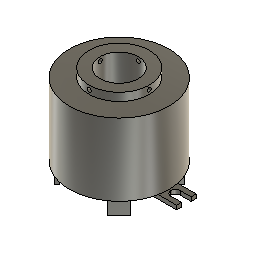
static base (Autodesk Fusion 360 archive; units mm, degrees)
design "slipring model"
Autodesk Fusion 360 part; units mm, degrees
sketch "Sketch1" plane through (0, 0, 0) normal (0, 0, 1) x (1, 0, 0)
  line L0 (36.0002, -9.75) -> (67.0101, -9.75)
  line L1 (67.0002, 9.75) -> (36.0002, 9.75)
  line L2 (67.0101, -4.75) -> (56.25, -4.75)
  arc A0 (56.25, 4.75) -> (51.5, 0) centre (56.25, 0) ccw
  line L3 (67.0101, -4.75) -> (67.0101, -9.75)
  line L4 (36.0002, 9.75) -> (36.0002, -9.75)
  arc A1 (51.5, 0) -> (56.25, -4.75) centre (56.25, 0) ccw
  line L5 (56.25, 4.75) -> (67.0002, 4.75)
  line L6 (67.0002, 4.75) -> (67.0002, 9.75)
  line L7 (0, 0) -> (36.0002, 0)
  point P0 (51.5001, 4.75)
  dimension "d7" = 4.75
  dimension "d8" = 4.75
  dimension "d9" = 4.75
  dimension "d10" = 31
  dimension "d11" = 19.5
  constraint perpendicular L5 L6
  constraint perpendicular L2 L3
  constraint tangent L2 A1
  constraint coincident P0 L5
  constraint tangent A0 L5
  constraint perpendicular L1 L6
  constraint perpendicular L1 L4
  constraint perpendicular L0 L3
  constraint coincident L7.start origin
  constraint midpoint L4 L7.end
  measures "d7" distance of A0.end P0
  measures "d8" radius of A1
  measures "d9" radius of A0
  measures "d10" distance of L1.start L1.end
  measures "d11" distance of L1.end L0.start
extrude "Extrude1" add sketch "Sketch1" along normal blind 4
sketch "Sketch2" plane through (0, 0, 4) normal (0, 0, 1) x (-1, 0, 0)
  line L0 (-56.25, -4.75) -> (-67.0002, -4.75)
  line L1 (-67.0002, -4.75) -> (-67.0002, -9.75)
  line L2 (-67.0101, 9.75) -> (-67.0101, 4.75)
  line L3 (-67.0101, 4.75) -> (-56.25, 4.75)
  arc A0 (-51.5, 0) -> (-56.25, 4.75) centre (-56.25, 0) ccw
  arc A1 (-56.25, -4.75) -> (-51.5, 0) centre (-56.25, 0) ccw
  circle A2 centre (0, 0) radius 49.5
  circle A3 centre (0, 0) radius 19.05
  dimension "d14" = 99
  dimension "d15" = 38.1
  constraint coincident A2.centre A3.centre
  measures "d14" diameter of A2
  measures "d15" diameter of A3
extrude "Extrude2" add sketch "Sketch2" along normal blind 72
sketch "Sketch3" plane through (0, 0, 76) normal (0, 0, 1) x (-1, 0, 0)
  circle A0 centre (0, 0) radius 19.05
  circle A1 centre (0, 0) radius 49.5
  circle A2 centre (0, 0) radius 19.05
  circle A3 centre (0, 0) radius 26
  constraint concentric A0 A2
  constraint concentric A2 A3
extrude "Extrude3" add sketch "Sketch3" along normal blind 0.5 contours A3
sketch "Sketch4" plane through (0, 0, 4) normal (0, 0, -1) x (1, 0, 0)
  line L0 (36.0002, 9.75) -> (48.5303, 9.75)
  arc A0 (48.5303, 9.75) -> (48.5303, -9.75) centre (0, 0) ccw
  line L1 (48.5303, -9.75) -> (36.0002, -9.75)
  line L2 (36.0002, -9.75) -> (36.0002, 9.75)
  circle A1 centre (0, 0) radius 19.05
  line L3 (0, 0) -> (39.0512, 0) construction
  line L4 (29.6134, 29.6134) -> (23.9565, 35.2703)
  line L5 (29.6134, 29.6134) -> (35.2703, 23.9565)
  line L6 (23.9565, 35.2703) -> (26.785, 38.0987)
  line L7 (35.2703, 23.9565) -> (38.0987, 26.785)
  line L8 (38.0987, 26.785) -> (26.785, 38.0987)
  line L9 (-29.6134, 29.6134) -> (-35.2703, 23.9565)
  line L10 (-35.2703, 23.9565) -> (-38.0987, 26.785)
  line L11 (-26.785, 38.0987) -> (-38.0987, 26.785)
  line L12 (-23.9565, 35.2703) -> (-26.785, 38.0987)
  line L13 (-29.6134, 29.6134) -> (-23.9565, 35.2703)
  line L14 (-29.6134, -29.6134) -> (-23.9565, -35.2703)
  line L15 (-23.9565, -35.2703) -> (-26.785, -38.0987)
  line L16 (-38.0987, -26.785) -> (-26.785, -38.0987)
  line L17 (-35.2703, -23.9565) -> (-38.0987, -26.785)
  line L18 (-29.6134, -29.6134) -> (-35.2703, -23.9565)
  line L19 (29.6134, -29.6134) -> (35.2703, -23.9565)
  line L20 (35.2703, -23.9565) -> (38.0987, -26.785)
  line L21 (26.785, -38.0987) -> (38.0987, -26.785)
  line L22 (23.9565, -35.2703) -> (26.785, -38.0987)
  line L23 (29.6134, -29.6134) -> (23.9565, -35.2703)
  dimension "d24" = 8
  dimension "d25" = 8
  dimension "d28" = 360
  constraint horizontal L3
  constraint coincident A0.centre A1.centre
  constraint perpendicular L4 L6
  constraint perpendicular L5 L7
  constraint perpendicular L6 L8
  measures "d24" distance of L4.start L4.end
  measures "d25" distance of L4.start L5.end
extrude "Extrude4" add sketch "Sketch4" along normal blind 15 contours L4 L5 L6 L7 L8 | L9 L10 L11 L12 L13 | L14 L15 L16 L17 L18 | L19 L20 L21 L22 L23
sketch "Sketch5" plane through (0, 0, 76.5) normal (0, 0, 1) x (-1, 0, 0)
  circle A0 centre (0, 0) radius 19.05
  circle A1 centre (0, 0) radius 30
  circle A2 centre (0, 0) radius 19.05
  dimension "d31" = 60
  constraint concentric A0 A1
  constraint coincident A0.centre A1.centre
  measures "d31" diameter of A1
extrude "Extrude5" add sketch "Sketch5" along normal blind 8
ref_plane "WorkPlane1" through (30, 0, 80.0207) normal (1, 0, 0) x (0, -1, 0)
sketch "Sketch6" plane through (30, 0, 0) normal (1, 0, 0) x (0, 1, 0)
  circle A0 centre (0, 80.5) radius 2
  dimension "d35" = 4
  measures "d35" diameter of A0
extrude "Extrude6" cut sketch "Sketch6" against normal blind 15.5
pattern_circular "C-Pattern1" count 4 over 360 about axis through (0, 0, 4) along (0, 0, 1) of "Extrude6"
equation "rotary_connect_length = 72 mm"
equation "d17 = rotary_connect_length"
equation "rotary_connect_space = 0.5 mm"
equation "rotary_connect_rotor_size = 8.5 mm"
equation "d21 = rotary_connect_space"
equation "d32 = rotary_connect_rotor_size - rotary_connect_space"
